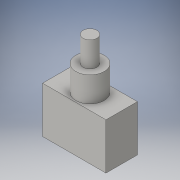
# Autodesk Inventor part: switch jp
Saved by Autodesk Inventor 2016 (Build 200138000, 138)
## iProperties
Created: 2017-09-11
Part Number: switch jp
Material: Generic
Document SubType Name: Modeling
Designer: student
Density: 1 g/cm^3
Appearance: Default
Author: student
Autodesk Inventor part; units mm, degrees
ref_plane "YZ Plane" through (0, 0, 0) normal (1, 0, 0) x (0, 1, 0)
ref_plane "XZ Plane" through (0, 0, 0) normal (0, 1, 0) x (-1, 0, 0)
ref_plane "XY Plane" through (0, 0, 0) normal (0, 0, 1) x (1, 0, 0)
sketch "Sketch1" plane through (0, 0, 0) normal (0, 0, 1) x (1, 0, 0)
  line L0 (-6.4008, -4.6609) -> (6.4008, -4.6609)
  line L1 (6.4008, -4.6609) -> (6.4008, 4.6609)
  line L2 (6.4008, 4.6609) -> (-6.4008, 4.6609)
  line L3 (-6.4008, 4.6609) -> (-6.4008, -4.6609)
  line L4 (-6.4008, -4.6609) -> (6.4008, 4.6609) construction
  line L5 (6.4008, -4.6609) -> (-6.4008, 4.6609) construction
  point P0 (0, 0)
  dimension "d0" = 12.8016
  dimension "d1" = 9.3218
  constraints: 12 end point, 2 midpoint, 2 parallel, 1 horizontal, 1 perpendicular
  measures "d0" distance between parallel lines of L1 L3
  measures "d1" distance of L0.end L1.end
extrude "Extrusion1" add sketch "Sketch1" along normal blind 6.35
sketch "Sketch2" plane through (-6.4008, 4.6609, 0) normal (0, 1, 0) x (1, 0, 0)
  line L0 (0, 0) -> (0, -6.35) projected
  line L1 (12.8016, 0) -> (12.8016, -6.35) projected
  line L2 (0, -6.35) -> (12.8016, -6.35) projected
  circle A0 centre (6.4008, -3.175) radius 2.8575
  point P0 (6.4008, 0)
  dimension "d4" = 5.715
  constraints: 1 centre point
  measures "d4" diameter of A0
extrude "Extrusion2" add sketch "Sketch2" along normal blind 5.08
sketch "Sketch3" plane through (0, 9.7409, 3.175) normal (0, 1, 0) x (1, 0, 0)
  circle A0 centre (0, 0) radius 1.397
  point P0 (0, 3.175)
  dimension "d7" = 2.794
  constraints: 1 centre point
  measures "d7" diameter of A0
extrude "Extrusion3" add sketch "Sketch3" along normal blind 5.08
body "Solid1"
